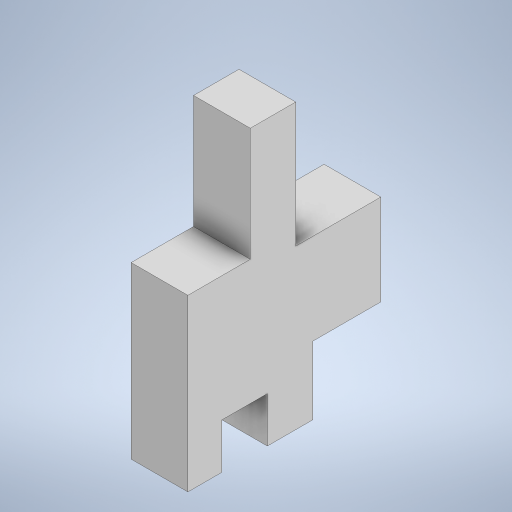
# Autodesk Inventor part: task3
Saved by Autodesk Inventor 2024.2 (Build 282272000, 272)
## iProperties
Created: 2024-10-18
Part Number: task3
Material: Типовые
Document SubType Name: Modeling
Designer: user
Density: 1 g/cm^3
Appearance: По умолчанию
Author: user
Autodesk Inventor part; units mm, degrees
ref_plane "YZ Plane" through (0, 0, 0) normal (1, 0, 0) x (0, 1, 0)
ref_plane "XZ Plane" through (0, 0, 0) normal (0, 1, 0) x (-1, 0, 0)
ref_plane "XY Plane" through (0, 0, 0) normal (0, 0, 1) x (1, 0, 0)
sketch "Эскиз1" plane through (0, 0, 0) normal (1, 0, 0) x (0, 1, 0)
  line L0 (0, -6) -> (0, -12)
  line L1 (0, -12) -> (8, -12)
  line L2 (8, -12) -> (8, -20)
  line L3 (8, -20) -> (0, -20)
  line L4 (0, -20) -> (0, -28)
  line L5 (0, -28) -> (12, -28)
  line L6 (12, -28) -> (12, -40)
  line L7 (12, -40) -> (28, -40)
  line L8 (28, -40) -> (28, -25)
  line L9 (28, -25) -> (50, -25)
  line L10 (50, -25) -> (50, -17)
  line L11 (50, -17) -> (30, -17)
  line L12 (30, -17) -> (30, -6)
  line L13 (30, -6) -> (0, -6)
  point P0 (0, 0)
  constraints: 28 end point, 10 perpendicular, 2 point on line, 1 horizontal, 1 vertical
extrude "Выдавливание1" add sketch "Эскиз1" along normal blind 10
